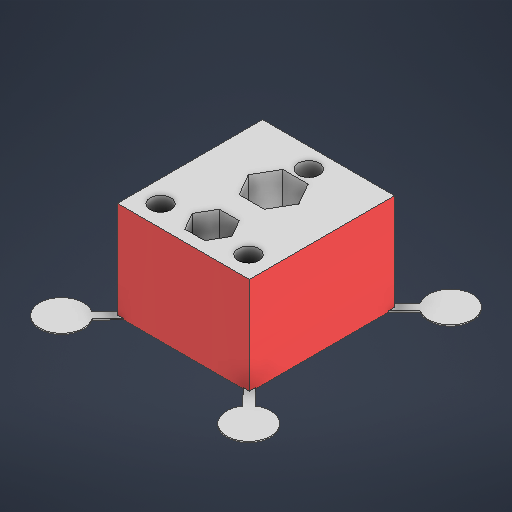
# Autodesk Inventor part: adapter-optical
Saved by Autodesk Inventor 2026.2 (Build 302298000, 298)
## iProperties
Created: 2026-05-22
Part Number: adapter-optical
Material: Generic
Document SubType Name: Modeling
Designer: mayhe
Density: 1 g/cm^3
Appearance: Default
Author: mayhe
Autodesk Inventor part; units mm, degrees
(part 1 of 2)
ref_plane "YZ Plane" through (0, 0, 0) normal (1, 0, 0) x (0, 1, 0)
ref_plane "XZ Plane" through (0, 0, 0) normal (0, 1, 0) x (-1, 0, 0)
ref_plane "XY Plane" through (0, 0, 0) normal (0, 0, 1) x (1, 0, 0)
sketch "Sketch1" plane through (0, 0, 0) normal (1, 0, 0) x (0, 1, 0)
  line L0 (11.125, 16.5) -> (-11.125, 16.5)
  line L1 (-11.125, 16.5) -> (-11.125, -16.5)
  line L2 (-11.125, -16.5) -> (11.125, -16.5)
  line L3 (11.125, -16.5) -> (11.125, 16.5)
  line L4 (11.125, 16.5) -> (-11.125, -16.5) construction
  line L5 (-11.125, 16.5) -> (11.125, -16.5) construction
  point P0 (0, 0)
  dimension "d0" = 22.25
  dimension "d1" = 33
  constraints: 12 end point, 2 midpoint, 2 parallel, 1 horizontal, 1 perpendicular
  measures "d0" distance of L2.end L1.end
  measures "d1" distance of L1.end L0.end
extrude "Extrusion1" add sketch "Sketch1" along normal mid plane 30
sketch "Sketch2" plane through (-15, -11.125, -16.5) normal (0, -1, 0) x (1, 0, 0)
  circle A0 centre (15, 4.5) radius 2.25
  line L0 (0, 0) -> (30, 0) projected
  circle A1 centre (25, 28.2) radius 2.25
  circle A2 centre (5, 28.2) radius 2.25
  point P0 (15, 16.5)
  dimension "d4" = 4.5
  dimension "d5" = 4.5
  dimension "d6" = 4.5
  dimension "d7" = 4.5
  dimension "d8" = 23.7
  dimension "d9" = 10
  dimension "d10" = 10
  constraints: 3 centre point, 1 horizontal alignment
  measures "d4" diameter of A0
  measures "d5" distance from line of L0 A0.centre
  measures "d6" diameter of A1
  measures "d7" diameter of A2
  measures "d8" vertical distance of A1.centre A0.centre
  measures "d9" horizontal distance of A0.centre A1.centre
  measures "d10" horizontal distance of A2.centre A0.centre
hole "Hole1" at (0, -11.125, -12) at (-10, -11.125, 11.7) at (10, -11.125, 11.7) direction (0, 1, 0) diameter 4.75 depth 22.25 tip angle 118 counterbore diameter 7.5 counterbore depth 3
sketch "Sketch4" plane through (-15, -11.125, -16.5) normal (0, -1, 0) x (1, 0, 0)
  circle A0 centre (15, 12.5) radius 2.0256
  circle A1 centre (15, 26.5) radius 2.1001
  line L0 (30, 33) -> (0, 33) projected
  point P0 (15, 16.5)
  point P1 (15, 33)
  dimension "d23" = 14
  dimension "d24" = 6.5
  constraints: 2 centre point, 1 midpoint
  measures "d23" distance of A1.centre A0.centre
  measures "d24" distance of point (15, 33) A1.centre
hole "Big Hole" at (0, -11.125, -4) direction (0, 1, 0) diameter 6.75 depth 22.25 tip angle 118
hole "Small Hole1" at (0, -11.125, 10) direction (0, 1, 0) diameter 5.75 depth 22.25 tip angle 118
sketch "Sketch5" plane through (-15, 11.125, 16.5) normal (0, 1, 0) x (1, 0, 0)
  circle A0 centre (15, 6.5) radius 2.875 projected
  circle A1 centre (15, 20.5) radius 3.375 projected
  circle A2 centre (15, 20.5) radius 4.975
  circle A3 centre (15, 6.5) radius 3.925
  line L0 (17.2661, 10.425) -> (19.5322, 6.5)
  line L1 (19.5322, 6.5) -> (17.2661, 2.575)
  line L2 (17.2661, 2.575) -> (12.7339, 2.575)
  line L3 (12.7339, 2.575) -> (10.4678, 6.5)
  line L4 (10.4678, 6.5) -> (12.7339, 10.425)
  line L5 (12.7339, 10.425) -> (17.2661, 10.425)
  line L6 (17.8723, 25.475) -> (20.7446, 20.5)
  line L7 (20.7446, 20.5) -> (17.8723, 15.525)
  line L8 (17.8723, 15.525) -> (12.1277, 15.525)
  line L9 (12.1277, 15.525) -> (9.2554, 20.5)
  line L10 (9.2554, 20.5) -> (12.1277, 25.475)
  line L11 (12.1277, 25.475) -> (17.8723, 25.475)
  point P0 (15, 16.5)
  point P1 (15, 10.425)
  point P2 (15, 25.475)
  dimension "d39" = 9.95
  dimension "d40" = 7.85
  constraints: 24 end point, 4 coincident, 2 midpoint, 2 vertical alignment, 30 other
extrude "Big nut seat" cut sketch "Sketch5" against normal blind 8.1168 contours A1 | A2 | A2 L6 L7 | A2 L11 L6 | L7 L8 A2 | A2 L10 L11 | L8 L9 A2 | A2 L9 L10
extrude "small nut seat" cut sketch "Sketch5" against normal blind 6.6168 contours A0 | A3 | A3 L0 L1 | A3 L5 L0 | L1 L2 A3 | A3 L4 L5 | L2 L3 A3 | A3 L3 L4
sketch "Sketch6" plane through (15, 11.125, -16.5) normal (0, 0, -1) x (-1, 0, 0)
  line L0 (2.368, -2.6371) -> (27.632, -2.6371) construction
  line L1 (27.632, -2.6371) -> (27.632, -19.6129) construction
  line L2 (27.632, -19.6129) -> (2.368, -19.6129) construction
  line L3 (2.368, -19.6129) -> (2.368, -2.6371) construction
  line L4 (12.625, 0) -> (17.375, 0) projected
  line L5 (15, 0) -> (15, -22.25)
  line L6 (17.875, -22.25) -> (12.125, -22.25) projected
  line L7 (30, 0) -> (0, 0) projected
  spline S0 degree 2 poles (11.0961, -2.1585) (11.269, -2.3611) (11.4617, -2.9539) (11.4617, -3.3343) knots 0 0 0 1 2 2 2
  spline S1 degree 2 poles (11.4617, -3.3343) (11.4617, -3.7048) (11.274, -4.305) (11.0961, -4.5075) knots 0 0 0 1 2 2 2
  spline S2 degree 2 poles (11.0961, -4.5075) (10.9084, -4.7199) (10.4119, -4.9225) (10.1131, -4.9225) knots 0 0 0 1 2 2 2
  spline S3 degree 2 poles (10.1131, -4.9225) (9.8043, -4.9225) (9.3103, -4.7125) (9.13, -4.5075) knots 0 0 0 1 2 2 2
  spline S4 degree 2 poles (9.13, -4.5075) (8.9546, -4.305) (8.7669, -3.7097) (8.7669, -3.3343) knots 0 0 0 1 2 2 2
  spline S5 degree 2 poles (8.7669, -3.3343) (8.7669, -2.9514) (8.9571, -2.3685) (9.1325, -2.1585) knots 0 0 0 1 2 2 2
  spline S6 degree 2 poles (9.1325, -2.1585) (9.3103, -1.956) (9.8068, -1.746) (10.1131, -1.746) knots 0 0 0 1 2 2 2
  spline S7 degree 2 poles (10.1131, -1.746) (10.4243, -1.746) (10.9232, -1.9634) (11.0961, -2.1585) knots 0 0 0 1 2 2 2
  spline S8 degree 2 poles (11.0393, -3.3343) (11.0393, -3.0329) (10.9084, -2.5661) (10.7899, -2.4129) knots 0 0 0 1 2 2 2
  spline S9 degree 2 poles (10.7899, -2.4129) (10.6688, -2.2549) (10.328, -2.0968) (10.1155, -2.0968) knots 0 0 0 1 2 2 2
  spline S10 degree 2 poles (10.1155, -2.0968) (9.8957, -2.0968) (9.5647, -2.2499) (9.4388, -2.4129) knots 0 0 0 1 2 2 2
  spline S11 degree 2 poles (9.4388, -2.4129) (9.3177, -2.5686) (9.1893, -3.0379) (9.1893, -3.3343) knots 0 0 0 1 2 2 2
  spline S12 degree 2 poles (9.1893, -3.3343) (9.1893, -3.9345) (9.6932, -4.5717) (10.1155, -4.5717) knots 0 0 0 1 2 2 2
  spline S13 degree 2 poles (10.1155, -4.5717) (10.5379, -4.5717) (11.0393, -3.9345) (11.0393, -3.3343) knots 0 0 0 1 2 2 2
  spline S14 degree 2 poles (13.7934, -3.6529) (13.7934, -4.2259) (13.2475, -4.9027) (12.8301, -4.9027) knots 0 0 0 1 2 2 2
  spline S15 degree 2 poles (12.8301, -4.9027) (12.6597, -4.9027) (12.3978, -4.8237) (12.262, -4.7422) knots 0 0 0 1 2 2 2
  line L8 (12.262, -4.7422) -> (12.262, -5.7005)
  line L9 (12.262, -5.7005) -> (11.8767, -5.7005)
  line L10 (11.8767, -5.7005) -> (11.8767, -2.571)
  line L11 (11.8767, -2.571) -> (12.262, -2.571)
  line L12 (12.262, -2.571) -> (12.262, -2.8106)
  spline S16 degree 2 poles (12.262, -2.8106) (12.4052, -2.6797) (12.756, -2.5068) (12.961, -2.5068) knots 0 0 0 1 2 2 2
  spline S17 degree 2 poles (12.961, -2.5068) (13.3537, -2.5068) (13.7934, -3.1293) (13.7934, -3.6529) knots 0 0 0 1 2 2 2
  spline S18 degree 2 poles (13.3957, -3.6974) (13.3957, -3.3046) (13.1463, -2.8724) (12.8671, -2.8724) knots 0 0 0 1 2 2 2
  spline S19 degree 2 poles (12.8671, -2.8724) (12.7041, -2.8724) (12.3978, -3.0181) (12.262, -3.1317) knots 0 0 0 1 2 2 2
  line L13 (12.262, -3.1317) -> (12.262, -4.431)
  spline S20 degree 2 poles (12.262, -4.431) (12.4127, -4.5026) (12.6275, -4.5569) (12.7659, -4.5569) knots 0 0 0 1 2 2 2
  spline S21 degree 2 poles (12.7659, -4.5569) (13.0647, -4.5569) (13.3957, -4.1173) (13.3957, -3.6974) knots 0 0 0 1 2 2 2
  spline S22 degree 2 poles (14.8851, -4.9027) (14.5715, -4.9027) (14.2182, -4.5446) (14.2182, -4.1568) knots 0 0 0 1 2 2 2
  line L14 (14.2182, -4.1568) -> (14.2182, -2.8897)
  line L15 (14.2182, -2.8897) -> (13.9589, -2.8897)
  line L16 (13.9589, -2.8897) -> (13.9589, -2.571)
  line L17 (13.9589, -2.571) -> (14.2182, -2.571)
  line L18 (14.2182, -2.571) -> (14.2182, -1.914)
  line L19 (14.2182, -1.914) -> (14.6036, -1.914)
  line L20 (14.6036, -1.914) -> (14.6036, -2.571)
  line L21 (14.6036, -2.571) -> (15.3125, -2.571)
  line L22 (15.3125, -2.571) -> (15.3125, -2.8897)
  line L23 (15.3125, -2.8897) -> (14.6036, -2.8897)
  line L24 (14.6036, -2.8897) -> (14.6036, -3.9789)
  spline S23 degree 2 poles (14.6036, -3.9789) (14.6036, -4.1518) (14.6159, -4.342) (14.6579, -4.4235) knots 0 0 0 1 2 2 2
  spline S24 degree 2 poles (14.6579, -4.4235) (14.6925, -4.4952) (14.8481, -4.5668) (14.9815, -4.5668) knots 0 0 0 1 2 2 2
  spline S25 degree 2 poles (14.9815, -4.5668) (15.0753, -4.5668) (15.2507, -4.51) (15.2902, -4.4927) knots 0 0 0 1 2 2 2
  line L25 (15.2902, -4.4927) -> (15.3125, -4.4927)
  line L26 (15.3125, -4.4927) -> (15.3125, -4.8385)
  spline S26 degree 2 poles (15.3125, -4.8385) (15.2038, -4.8681) (14.9815, -4.9027) (14.8851, -4.9027) knots 0 0 0 1 2 2 2
  line L27 (15.9892, -4.8583) -> (15.6039, -4.8583)
  line L28 (15.6039, -4.8583) -> (15.6039, -2.571)
  line L29 (15.6039, -2.571) -> (15.9892, -2.571)
  line L30 (15.9892, -2.571) -> (15.9892, -4.8583)
  line L31 (16.0164, -2.1906) -> (15.5792, -2.1906)
  line L32 (15.5792, -2.1906) -> (15.5792, -1.7905)
  line L33 (15.5792, -1.7905) -> (16.0164, -1.7905)
  line L34 (16.0164, -1.7905) -> (16.0164, -2.1906)
  spline S27 degree 2 poles (17.4638, -4.9101) (17.2267, -4.9101) (16.834, -4.7644) (16.6932, -4.6162) knots 0 0 0 1 2 2 2
  spline S28 degree 2 poles (16.6932, -4.6162) (16.5524, -4.4705) (16.3968, -4.0209) (16.3968, -3.7196) knots 0 0 0 1 2 2 2
  spline S29 degree 2 poles (16.3968, -3.7196) (16.3968, -3.4182) (16.5573, -2.9786) (16.6932, -2.8304) knots 0 0 0 1 2 2 2
  spline S30 degree 2 poles (16.6932, -2.8304) (16.829, -2.6797) (17.2317, -2.5192) (17.4638, -2.5192) knots 0 0 0 1 2 2 2
  spline S31 degree 2 poles (17.4638, -2.5192) (17.6516, -2.5192) (18.0023, -2.6254) (18.1382, -2.6945) knots 0 0 0 1 2 2 2
  line L35 (18.1382, -2.6945) -> (18.1382, -3.1268)
  line L36 (18.1382, -3.1268) -> (18.1159, -3.1268)
  spline S32 degree 2 poles (18.1159, -3.1268) (18.0739, -3.0922) (17.9455, -3.0033) (17.8541, -2.9564) knots 0 0 0 1 2 2 2
  spline S33 degree 2 poles (17.8541, -2.9564) (17.7726, -2.9168) (17.5552, -2.8551) (17.4564, -2.8551) knots 0 0 0 1 2 2 2
  spline S34 degree 2 poles (17.4564, -2.8551) (17.1576, -2.8551) (16.7945, -3.3071) (16.7945, -3.7196) knots 0 0 0 1 2 2 2
  spline S35 degree 2 poles (16.7945, -3.7196) (16.7945, -4.1222) (17.1452, -4.5742) (17.4564, -4.5742) knots 0 0 0 1 2 2 2
  spline S36 degree 2 poles (17.4564, -4.5742) (17.6442, -4.5742) (17.985, -4.4186) (18.1159, -4.2976) knots 0 0 0 1 2 2 2
  line L37 (18.1159, -4.2976) -> (18.1382, -4.2976)
  line L38 (18.1382, -4.2976) -> (18.1382, -4.7298)
  spline S37 degree 2 poles (18.1382, -4.7298) (18.0813, -4.757) (17.9084, -4.8336) (17.8393, -4.8509) knots 0 0 0 1 2 2 2
  spline S38 degree 2 poles (17.8393, -4.8509) (17.7405, -4.8805) (17.5849, -4.9101) (17.4638, -4.9101) knots 0 0 0 1 2 2 2
  spline S39 degree 2 poles (19.7634, -4.6162) (19.7165, -4.6508) (19.5584, -4.7743) (19.4843, -4.8113) knots 0 0 0 1 2 2 2
  spline S40 degree 2 poles (19.4843, -4.8113) (19.383, -4.8657) (19.1929, -4.9225) (19.02, -4.9225) knots 0 0 0 1 2 2 2
  spline S41 degree 2 poles (19.02, -4.9225) (18.8792, -4.9225) (18.6247, -4.8163) (18.5284, -4.7199) knots 0 0 0 1 2 2 2
  spline S42 degree 2 poles (18.5284, -4.7199) (18.437, -4.6261) (18.3259, -4.3494) (18.3259, -4.1963) knots 0 0 0 1 2 2 2
  spline S43 degree 2 poles (18.3259, -4.1963) (18.3259, -3.9592) (18.5259, -3.6233) (18.7433, -3.5269) knots 0 0 0 1 2 2 2
  spline S44 degree 2 poles (18.7433, -3.5269) (18.936, -3.438) (19.4596, -3.3713) (19.7634, -3.354) knots 0 0 0 1 2 2 2
  line L39 (19.7634, -3.354) -> (19.7634, -3.2799)
  spline S45 degree 2 poles (19.7634, -3.2799) (19.7634, -3.1465) (19.6819, -2.9811) (19.6078, -2.9341) knots 0 0 0 1 2 2 2
  spline S46 degree 2 poles (19.6078, -2.9341) (19.5337, -2.8872) (19.3213, -2.8576) (19.2077, -2.8576) knots 0 0 0 1 2 2 2
  spline S47 degree 2 poles (19.2077, -2.8576) (19.0743, -2.8576) (18.7137, -2.9366) (18.5334, -3.0132) knots 0 0 0 1 2 2 2
  line L40 (18.5334, -3.0132) -> (18.5111, -3.0132)
  line L41 (18.5111, -3.0132) -> (18.5111, -2.6204)
  spline S48 degree 2 poles (18.5111, -2.6204) (18.6173, -2.5908) (19.015, -2.5167) (19.2101, -2.5167) knots 0 0 0 1 2 2 2
  spline S49 degree 2 poles (19.2101, -2.5167) (19.4473, -2.5167) (19.7708, -2.5908) (19.8993, -2.6871) knots 0 0 0 1 2 2 2
  spline S50 degree 2 poles (19.8993, -2.6871) (20.0252, -2.781) (20.1487, -3.0799) (20.1487, -3.2947) knots 0 0 0 1 2 2 2
  line L42 (20.1487, -3.2947) -> (20.1487, -4.8583)
  line L43 (20.1487, -4.8583) -> (19.7634, -4.8583)
  line L44 (19.7634, -4.8583) -> (19.7634, -4.6162)
  line L45 (19.7634, -4.2951) -> (19.7634, -3.6603)
  spline S51 degree 2 poles (19.7634, -3.6603) (19.6251, -3.6727) (19.2077, -3.7146) (19.0768, -3.7542) knots 0 0 0 1 2 2 2
  spline S52 degree 2 poles (19.0768, -3.7542) (18.9236, -3.8011) (18.7235, -3.9962) (18.7235, -4.1691) knots 0 0 0 1 2 2 2
  spline S53 degree 2 poles (18.7235, -4.1691) (18.7235, -4.3667) (18.9459, -4.5668) (19.1583, -4.5668) knots 0 0 0 1 2 2 2
  spline S54 degree 2 poles (19.1583, -4.5668) (19.3386, -4.5668) (19.635, -4.4112) (19.7634, -4.2951) knots 0 0 0 1 2 2 2
  line L46 (21.0824, -4.8583) -> (20.6971, -4.8583)
  line L47 (20.6971, -4.8583) -> (20.6971, -1.6744)
  line L48 (20.6971, -1.6744) -> (21.0824, -1.6744)
  line L49 (21.0824, -1.6744) -> (21.0824, -4.8583)
  spline S55 degree 2 poles (9.4215, -9.9311) (9.1251, -9.9311) (8.6237, -9.731) (8.4409, -9.5309) knots 0 0 0 1 2 2 2
  spline S56 degree 2 poles (8.4409, -9.5309) (8.2581, -9.3333) (8.058, -8.7405) (8.058, -8.3552) knots 0 0 0 1 2 2 2
  spline S57 degree 2 poles (8.058, -8.3552) (8.058, -7.9723) (8.2532, -7.4042) (8.4384, -7.1943) knots 0 0 0 1 2 2 2
  spline S58 degree 2 poles (8.4384, -7.1943) (8.6212, -6.9893) (9.1201, -6.7744) (9.4289, -6.7744) knots 0 0 0 1 2 2 2
  spline S59 degree 2 poles (9.4289, -6.7744) (9.582, -6.7744) (9.8513, -6.8188) (9.9649, -6.8534) knots 0 0 0 1 2 2 2
  spline S60 degree 2 poles (9.9649, -6.8534) (10.0637, -6.8855) (10.2687, -6.9769) (10.37, -7.0313) knots 0 0 0 1 2 2 2
  line L50 (10.37, -7.0313) -> (10.37, -7.5203)
  line L51 (10.37, -7.5203) -> (10.3378, -7.5203)
  spline S61 degree 2 poles (10.3378, -7.5203) (10.2835, -7.4709) (10.1155, -7.3326) (9.9945, -7.2659) knots 0 0 0 1 2 2 2
  spline S62 degree 2 poles (9.9945, -7.2659) (9.8784, -7.2017) (9.6042, -7.1202) (9.4264, -7.1202) knots 0 0 0 1 2 2 2
  spline S63 degree 2 poles (9.4264, -7.1202) (9.2313, -7.1202) (8.883, -7.2807) (8.7521, -7.4339) knots 0 0 0 1 2 2 2
  spline S64 degree 2 poles (8.7521, -7.4339) (8.6237, -7.5895) (8.4804, -8.0613) (8.4804, -8.3552) knots 0 0 0 1 2 2 2
  spline S65 degree 2 poles (8.4804, -8.3552) (8.4804, -8.6689) (8.6311, -9.1209) (8.762, -9.2765) knots 0 0 0 1 2 2 2
  spline S66 degree 2 poles (8.762, -9.2765) (8.8904, -9.4272) (9.2337, -9.5803) (9.4264, -9.5803) knots 0 0 0 1 2 2 2
  spline S67 degree 2 poles (9.4264, -9.5803) (9.6018, -9.5803) (9.9007, -9.4939) (10.0167, -9.4296) knots 0 0 0 1 2 2 2
  spline S68 degree 2 poles (10.0167, -9.4296) (10.1279, -9.3654) (10.2934, -9.232) (10.3403, -9.1851) knots 0 0 0 1 2 2 2
  line L52 (10.3403, -9.1851) -> (10.37, -9.1851)
  line L53 (10.37, -9.1851) -> (10.37, -9.6692)
  spline S69 degree 2 poles (10.37, -9.6692) (10.2687, -9.7162) (10.0908, -9.8026) (9.9649, -9.8421) knots 0 0 0 1 2 2 2
  spline S70 degree 2 poles (9.9649, -9.8421) (9.8315, -9.8866) (9.6042, -9.9311) (9.4215, -9.9311) knots 0 0 0 1 2 2 2
  spline S71 degree 2 poles (11.9928, -9.6347) (11.9458, -9.6692) (11.7877, -9.7927) (11.7136, -9.8298) knots 0 0 0 1 2 2 2
  spline S72 degree 2 poles (11.7136, -9.8298) (11.6124, -9.8841) (11.4222, -9.9409) (11.2493, -9.9409) knots 0 0 0 1 2 2 2
  spline S73 degree 2 poles (11.2493, -9.9409) (11.1085, -9.9409) (10.8541, -9.8347) (10.7577, -9.7384) knots 0 0 0 1 2 2 2
  spline S74 degree 2 poles (10.7577, -9.7384) (10.6664, -9.6445) (10.5552, -9.3679) (10.5552, -9.2148) knots 0 0 0 1 2 2 2
  spline S75 degree 2 poles (10.5552, -9.2148) (10.5552, -8.9776) (10.7553, -8.6417) (10.9726, -8.5454) knots 0 0 0 1 2 2 2
  spline S76 degree 2 poles (10.9726, -8.5454) (11.1653, -8.4565) (11.6889, -8.3898) (11.9928, -8.3725) knots 0 0 0 1 2 2 2
  line L54 (11.9928, -8.3725) -> (11.9928, -8.2984)
  spline S77 degree 2 poles (11.9928, -8.2984) (11.9928, -8.165) (11.9112, -7.9995) (11.8371, -7.9526) knots 0 0 0 1 2 2 2
  spline S78 degree 2 poles (11.8371, -7.9526) (11.763, -7.9056) (11.5506, -7.876) (11.437, -7.876) knots 0 0 0 1 2 2 2
  spline S79 degree 2 poles (11.437, -7.876) (11.3036, -7.876) (10.943, -7.955) (10.7627, -8.0316) knots 0 0 0 1 2 2 2
  line L55 (10.7627, -8.0316) -> (10.7405, -8.0316)
  line L56 (10.7405, -8.0316) -> (10.7405, -7.6389)
  spline S80 degree 2 poles (10.7405, -7.6389) (10.8467, -7.6092) (11.2443, -7.5351) (11.4395, -7.5351) knots 0 0 0 1 2 2 2
  spline S81 degree 2 poles (11.4395, -7.5351) (11.6766, -7.5351) (12.0002, -7.6092) (12.1286, -7.7056) knots 0 0 0 1 2 2 2
  spline S82 degree 2 poles (12.1286, -7.7056) (12.2546, -7.7994) (12.3781, -8.0983) (12.3781, -8.3132) knots 0 0 0 1 2 2 2
  line L57 (12.3781, -8.3132) -> (12.3781, -9.8767)
  line L58 (12.3781, -9.8767) -> (11.9928, -9.8767)
  line L59 (11.9928, -9.8767) -> (11.9928, -9.6347)
  line L60 (11.9928, -9.3136) -> (11.9928, -8.6788)
  spline S83 degree 2 poles (11.9928, -8.6788) (11.8544, -8.6911) (11.437, -8.7331) (11.3061, -8.7726) knots 0 0 0 1 2 2 2
  spline S84 degree 2 poles (11.3061, -8.7726) (11.1529, -8.8196) (10.9529, -9.0147) (10.9529, -9.1876) knots 0 0 0 1 2 2 2
  spline S85 degree 2 poles (10.9529, -9.1876) (10.9529, -9.3852) (11.1752, -9.5853) (11.3876, -9.5853) knots 0 0 0 1 2 2 2
  spline S86 degree 2 poles (11.3876, -9.5853) (11.5679, -9.5853) (11.8643, -9.4296) (11.9928, -9.3136) knots 0 0 0 1 2 2 2
  line L61 (15.5125, -9.8767) -> (15.5125, -8.5528)
  spline S87 degree 2 poles (15.5125, -8.5528) (15.5125, -8.3947) (15.4878, -8.1255) (15.4483, -8.0514) knots 0 0 0 1 2 2 2
  spline S88 degree 2 poles (15.4483, -8.0514) (15.4088, -7.9699) (15.2581, -7.8908) (15.1272, -7.8908) knots 0 0 0 1 2 2 2
  spline S89 degree 2 poles (15.1272, -7.8908) (15.0086, -7.8908) (14.7369, -8.0366) (14.5937, -8.1749) knots 0 0 0 1 2 2 2
  spline S90 degree 2 poles (14.5937, -8.1749) (14.5962, -8.2095) (14.6011, -8.3058) (14.6011, -8.37) knots 0 0 0 1 2 2 2
  line L62 (14.6011, -8.37) -> (14.6011, -9.8767)
  line L63 (14.6011, -9.8767) -> (14.2158, -9.8767)
  line L64 (14.2158, -9.8767) -> (14.2158, -8.5528)
  spline S91 degree 2 poles (14.2158, -8.5528) (14.2158, -8.3947) (14.1911, -8.1255) (14.1515, -8.0514) knots 0 0 0 1 2 2 2
  spline S92 degree 2 poles (14.1515, -8.0514) (14.112, -7.9699) (13.9614, -7.8908) (13.8304, -7.8908) knots 0 0 0 1 2 2 2
  spline S93 degree 2 poles (13.8304, -7.8908) (13.7069, -7.8908) (13.4328, -8.0464) (13.3043, -8.1675) knots 0 0 0 1 2 2 2
  line L65 (13.3043, -8.1675) -> (13.3043, -9.8767)
  line L66 (13.3043, -9.8767) -> (12.919, -9.8767)
  line L67 (12.919, -9.8767) -> (12.919, -7.5895)
  line L68 (12.919, -7.5895) -> (13.3043, -7.5895)
  line L69 (13.3043, -7.5895) -> (13.3043, -7.8414)
  spline S94 degree 2 poles (13.3043, -7.8414) (13.455, -7.6908) (13.7514, -7.5253) (13.9292, -7.5253) knots 0 0 0 1 2 2 2
  spline S95 degree 2 poles (13.9292, -7.5253) (14.1318, -7.5253) (14.4455, -7.7105) (14.527, -7.9205) knots 0 0 0 1 2 2 2
  spline S96 degree 2 poles (14.527, -7.9205) (14.7024, -7.7253) (15.0333, -7.5253) (15.226, -7.5253) knots 0 0 0 1 2 2 2
  spline S97 degree 2 poles (15.226, -7.5253) (15.3742, -7.5253) (15.6163, -7.6167) (15.7052, -7.7204) knots 0 0 0 1 2 2 2
  spline S98 degree 2 poles (15.7052, -7.7204) (15.7966, -7.8241) (15.8979, -8.1354) (15.8979, -8.37) knots 0 0 0 1 2 2 2
  line L70 (15.8979, -8.37) -> (15.8979, -9.8767)
  line L71 (15.8979, -9.8767) -> (15.5125, -9.8767)
  spline S99 degree 2 poles (17.4317, -9.9286) (16.8834, -9.9286) (16.2807, -9.3136) (16.2807, -8.7454) knots 0 0 0 1 2 2 2
  spline S100 degree 2 poles (16.2807, -8.7454) (16.2807, -8.1872) (16.8661, -7.5253) (17.3379, -7.5253) knots 0 0 0 1 2 2 2
  spline S101 degree 2 poles (17.3379, -7.5253) (17.5503, -7.5253) (17.8788, -7.6488) (17.9998, -7.7797) knots 0 0 0 1 2 2 2
  spline S102 degree 2 poles (17.9998, -7.7797) (18.1233, -7.9106) (18.2542, -8.2885) (18.2542, -8.5627) knots 0 0 0 1 2 2 2
  line L72 (18.2542, -8.5627) -> (18.2542, -8.7726)
  line L73 (18.2542, -8.7726) -> (16.671, -8.7726)
  spline S103 degree 2 poles (16.671, -8.7726) (16.671, -9.1703) (17.0711, -9.5927) (17.4268, -9.5927) knots 0 0 0 1 2 2 2
  spline S104 degree 2 poles (17.4268, -9.5927) (17.5528, -9.5927) (17.7973, -9.5359) (17.8961, -9.4914) knots 0 0 0 1 2 2 2
  spline S105 degree 2 poles (17.8961, -9.4914) (17.9998, -9.442) (18.1431, -9.3555) (18.19, -9.316) knots 0 0 0 1 2 2 2
  line L74 (18.19, -9.316) -> (18.2123, -9.316)
  line L75 (18.2123, -9.316) -> (18.2123, -9.7359)
  spline S106 degree 2 poles (18.2123, -9.7359) (18.1456, -9.7631) (17.943, -9.8421) (17.864, -9.8644) knots 0 0 0 1 2 2 2
  spline S107 degree 2 poles (17.864, -9.8644) (17.7528, -9.8965) (17.5701, -9.9286) (17.4317, -9.9286) knots 0 0 0 1 2 2 2
  spline S108 degree 2 poles (17.8788, -8.4787) (17.8739, -8.3231) (17.8096, -8.0958) (17.7479, -8.0193) knots 0 0 0 1 2 2 2
  spline S109 degree 2 poles (17.7479, -8.0193) (17.6812, -7.9328) (17.4713, -7.8414) (17.3156, -7.8414) knots 0 0 0 1 2 2 2
  spline S110 degree 2 poles (17.3156, -7.8414) (17.1625, -7.8414) (16.9476, -7.9328) (16.8587, -8.0217) knots 0 0 0 1 2 2 2
  spline S111 degree 2 poles (16.8587, -8.0217) (16.7722, -8.1131) (16.6833, -8.333) (16.671, -8.4787) knots 0 0 0 1 2 2 2
  line L76 (16.671, -8.4787) -> (17.8788, -8.4787)
  line L77 (19.8573, -8.002) -> (19.8375, -8.002)
  spline S112 degree 2 poles (19.8375, -8.002) (19.7931, -7.9896) (19.6967, -7.9847) (19.63, -7.9847) knots 0 0 0 1 2 2 2
  spline S113 degree 2 poles (19.63, -7.9847) (19.4744, -7.9847) (19.1682, -8.1205) (19.0298, -8.2539) knots 0 0 0 1 2 2 2
  line L78 (19.0298, -8.2539) -> (19.0298, -9.8767)
  line L79 (19.0298, -9.8767) -> (18.6445, -9.8767)
  line L80 (18.6445, -9.8767) -> (18.6445, -7.5895)
  line L81 (18.6445, -7.5895) -> (19.0298, -7.5895)
  line L82 (19.0298, -7.5895) -> (19.0298, -7.9303)
  spline S114 degree 2 poles (19.0298, -7.9303) (19.2398, -7.7426) (19.5535, -7.5895) (19.7017, -7.5895) knots 0 0 0 1 2 2 2
  spline S115 degree 2 poles (19.7017, -7.5895) (19.761, -7.5895) (19.8202, -7.5944) (19.8573, -7.6018) knots 0 0 0 1 2 2 2
  line L83 (19.8573, -7.6018) -> (19.8573, -8.002)
  spline S116 degree 2 poles (21.4307, -9.6347) (21.3838, -9.6692) (21.2257, -9.7927) (21.1516, -9.8298) knots 0 0 0 1 2 2 2
  spline S117 degree 2 poles (21.1516, -9.8298) (21.0503, -9.8841) (20.8601, -9.9409) (20.6872, -9.9409) knots 0 0 0 1 2 2 2
  spline S118 degree 2 poles (20.6872, -9.9409) (20.5464, -9.9409) (20.292, -9.8347) (20.1957, -9.7384) knots 0 0 0 1 2 2 2
  spline S119 degree 2 poles (20.1957, -9.7384) (20.1043, -9.6445) (19.9931, -9.3679) (19.9931, -9.2148) knots 0 0 0 1 2 2 2
  spline S120 degree 2 poles (19.9931, -9.2148) (19.9931, -8.9776) (20.1932, -8.6417) (20.4106, -8.5454) knots 0 0 0 1 2 2 2
  spline S121 degree 2 poles (20.4106, -8.5454) (20.6032, -8.4565) (21.1269, -8.3898) (21.4307, -8.3725) knots 0 0 0 1 2 2 2
  line L84 (21.4307, -8.3725) -> (21.4307, -8.2984)
  spline S122 degree 2 poles (21.4307, -8.2984) (21.4307, -8.165) (21.3492, -7.9995) (21.2751, -7.9526) knots 0 0 0 1 2 2 2
  spline S123 degree 2 poles (21.2751, -7.9526) (21.201, -7.9056) (20.9886, -7.876) (20.8749, -7.876) knots 0 0 0 1 2 2 2
  spline S124 degree 2 poles (20.8749, -7.876) (20.7416, -7.876) (20.3809, -7.955) (20.2006, -8.0316) knots 0 0 0 1 2 2 2
  line L85 (20.2006, -8.0316) -> (20.1784, -8.0316)
  line L86 (20.1784, -8.0316) -> (20.1784, -7.6389)
  spline S125 degree 2 poles (20.1784, -7.6389) (20.2846, -7.6092) (20.6823, -7.5351) (20.8774, -7.5351) knots 0 0 0 1 2 2 2
  spline S126 degree 2 poles (20.8774, -7.5351) (21.1145, -7.5351) (21.4381, -7.6092) (21.5665, -7.7056) knots 0 0 0 1 2 2 2
  spline S127 degree 2 poles (21.5665, -7.7056) (21.6925, -7.7994) (21.816, -8.0983) (21.816, -8.3132) knots 0 0 0 1 2 2 2
  line L87 (21.816, -8.3132) -> (21.816, -9.8767)
  line L88 (21.816, -9.8767) -> (21.4307, -9.8767)
  line L89 (21.4307, -9.8767) -> (21.4307, -9.6347)
  line L90 (21.4307, -9.3136) -> (21.4307, -8.6788)
  spline S128 degree 2 poles (21.4307, -8.6788) (21.2924, -8.6911) (20.8749, -8.7331) (20.744, -8.7726) knots 0 0 0 1 2 2 2
  spline S129 degree 2 poles (20.744, -8.7726) (20.5909, -8.8196) (20.3908, -9.0147) (20.3908, -9.1876) knots 0 0 0 1 2 2 2
  spline S130 degree 2 poles (20.3908, -9.1876) (20.3908, -9.3852) (20.6131, -9.5853) (20.8255, -9.5853) knots 0 0 0 1 2 2 2
  spline S131 degree 2 poles (20.8255, -9.5853) (21.0058, -9.5853) (21.3022, -9.4296) (21.4307, -9.3136) knots 0 0 0 1 2 2 2
  line L91 (7.7456, -14.8952) -> (8.7731, -11.8472)
  line L92 (8.7731, -11.8472) -> (9.272, -11.8472)
  line L93 (9.272, -11.8472) -> (10.2996, -14.8952)
  line L94 (10.2996, -14.8952) -> (9.8722, -14.8952)
  line L95 (9.8722, -14.8952) -> (9.5956, -14.043)
  line L96 (9.5956, -14.043) -> (8.4322, -14.043)
  line L97 (8.4322, -14.043) -> (8.1556, -14.8952)
  line L98 (8.1556, -14.8952) -> (7.7456, -14.8952)
  line L99 (9.4845, -13.6972) -> (9.0127, -12.2621)
  line L100 (9.0127, -12.2621) -> (8.5434, -13.6972)
  line L101 (8.5434, -13.6972) -> (9.4845, -13.6972)
  line L102 (12.3176, -14.8952) -> (11.9322, -14.8952)
  line L103 (11.9322, -14.8952) -> (11.9322, -14.663)
  spline S132 degree 2 poles (11.9322, -14.663) (11.8433, -14.7371) (11.7124, -14.8359) (11.6235, -14.8779) knots 0 0 0 1 2 2 2
  spline S133 degree 2 poles (11.6235, -14.8779) (11.542, -14.9174) (11.3666, -14.9594) (11.2505, -14.9594) knots 0 0 0 1 2 2 2
  spline S134 degree 2 poles (11.2505, -14.9594) (11.0628, -14.9594) (10.7466, -14.8038) (10.6355, -14.6531) knots 0 0 0 1 2 2 2
  spline S135 degree 2 poles (10.6355, -14.6531) (10.5243, -14.5024) (10.4008, -14.0578) (10.4008, -13.7688) knots 0 0 0 1 2 2 2
  spline S136 degree 2 poles (10.4008, -13.7688) (10.4008, -13.4675) (10.5564, -13.0278) (10.6923, -12.8623) knots 0 0 0 1 2 2 2
  spline S137 degree 2 poles (10.6923, -12.8623) (10.8183, -12.7141) (11.1715, -12.5437) (11.3666, -12.5437) knots 0 0 0 1 2 2 2
  spline S138 degree 2 poles (11.3666, -12.5437) (11.537, -12.5437) (11.7914, -12.6203) (11.9322, -12.6993) knots 0 0 0 1 2 2 2
  line L104 (11.9322, -12.6993) -> (11.9322, -11.7113)
  line L105 (11.9322, -11.7113) -> (12.3176, -11.7113)
  line L106 (12.3176, -11.7113) -> (12.3176, -14.8952)
  line L107 (11.9322, -14.3394) -> (11.9322, -13.018)
  spline S139 degree 2 poles (11.9322, -13.018) (11.789, -12.9488) (11.5617, -12.8969) (11.4308, -12.8969) knots 0 0 0 1 2 2 2
  spline S140 degree 2 poles (11.4308, -12.8969) (11.1344, -12.8969) (10.7985, -13.3415) (10.7985, -13.7614) knots 0 0 0 1 2 2 2
  spline S141 degree 2 poles (10.7985, -13.7614) (10.7985, -14.1665) (11.0554, -14.5938) (11.3394, -14.5938) knots 0 0 0 1 2 2 2
  spline S142 degree 2 poles (11.3394, -14.5938) (11.4901, -14.5938) (11.7964, -14.4555) (11.9322, -14.3394) knots 0 0 0 1 2 2 2
  spline S143 degree 2 poles (14.1503, -14.6531) (14.1034, -14.6877) (13.9453, -14.8112) (13.8712, -14.8482) knots 0 0 0 1 2 2 2
  spline S144 degree 2 poles (13.8712, -14.8482) (13.7699, -14.9026) (13.5797, -14.9594) (13.4068, -14.9594) knots 0 0 0 1 2 2 2
  spline S145 degree 2 poles (13.4068, -14.9594) (13.266, -14.9594) (13.0116, -14.8532) (12.9153, -14.7568) knots 0 0 0 1 2 2 2
  spline S146 degree 2 poles (12.9153, -14.7568) (12.8239, -14.663) (12.7128, -14.3863) (12.7128, -14.2332) knots 0 0 0 1 2 2 2
  spline S147 degree 2 poles (12.7128, -14.2332) (12.7128, -13.9961) (12.9128, -13.6602) (13.1302, -13.5638) knots 0 0 0 1 2 2 2
  spline S148 degree 2 poles (13.1302, -13.5638) (13.3229, -13.4749) (13.8465, -13.4082) (14.1503, -13.3909) knots 0 0 0 1 2 2 2
  line L108 (14.1503, -13.3909) -> (14.1503, -13.3168)
  spline S149 degree 2 poles (14.1503, -13.3168) (14.1503, -13.1834) (14.0688, -13.018) (13.9947, -12.971) knots 0 0 0 1 2 2 2
  spline S150 degree 2 poles (13.9947, -12.971) (13.9206, -12.9241) (13.7082, -12.8945) (13.5946, -12.8945) knots 0 0 0 1 2 2 2
  spline S151 degree 2 poles (13.5946, -12.8945) (13.4612, -12.8945) (13.1006, -12.9735) (12.9202, -13.0501) knots 0 0 0 1 2 2 2
  line L109 (12.9202, -13.0501) -> (12.898, -13.0501)
  line L110 (12.898, -13.0501) -> (12.898, -12.6573)
  spline S152 degree 2 poles (12.898, -12.6573) (13.0042, -12.6277) (13.4019, -12.5536) (13.597, -12.5536) knots 0 0 0 1 2 2 2
  spline S153 degree 2 poles (13.597, -12.5536) (13.8342, -12.5536) (14.1577, -12.6277) (14.2862, -12.724) knots 0 0 0 1 2 2 2
  spline S154 degree 2 poles (14.2862, -12.724) (14.4121, -12.8179) (14.5356, -13.1168) (14.5356, -13.3316) knots 0 0 0 1 2 2 2
  line L111 (14.5356, -13.3316) -> (14.5356, -14.8952)
  line L112 (14.5356, -14.8952) -> (14.1503, -14.8952)
  line L113 (14.1503, -14.8952) -> (14.1503, -14.6531)
  line L114 (14.1503, -14.332) -> (14.1503, -13.6972)
  spline S155 degree 2 poles (14.1503, -13.6972) (14.012, -13.7096) (13.5946, -13.7516) (13.4636, -13.7911) knots 0 0 0 1 2 2 2
  spline S156 degree 2 poles (13.4636, -13.7911) (13.3105, -13.838) (13.1104, -14.0331) (13.1104, -14.206) knots 0 0 0 1 2 2 2
  spline S157 degree 2 poles (13.1104, -14.206) (13.1104, -14.4036) (13.3327, -14.6037) (13.5452, -14.6037) knots 0 0 0 1 2 2 2
  spline S158 degree 2 poles (13.5452, -14.6037) (13.7255, -14.6037) (14.0219, -14.4481) (14.1503, -14.332) knots 0 0 0 1 2 2 2
  spline S159 degree 2 poles (16.9933, -13.6898) (16.9933, -14.2628) (16.4474, -14.9396) (16.03, -14.9396) knots 0 0 0 1 2 2 2
  spline S160 degree 2 poles (16.03, -14.9396) (15.8596, -14.9396) (15.5977, -14.8606) (15.4619, -14.7791) knots 0 0 0 1 2 2 2
  line L115 (15.4619, -14.7791) -> (15.4619, -15.7374)
  line L116 (15.4619, -15.7374) -> (15.0766, -15.7374)
  line L117 (15.0766, -15.7374) -> (15.0766, -12.6079)
  line L118 (15.0766, -12.6079) -> (15.4619, -12.6079)
  line L119 (15.4619, -12.6079) -> (15.4619, -12.8475)
  spline S161 degree 2 poles (15.4619, -12.8475) (15.6052, -12.7166) (15.9559, -12.5437) (16.1609, -12.5437) knots 0 0 0 1 2 2 2
  spline S162 degree 2 poles (16.1609, -12.5437) (16.5536, -12.5437) (16.9933, -13.1662) (16.9933, -13.6898) knots 0 0 0 1 2 2 2
  spline S163 degree 2 poles (16.5956, -13.7343) (16.5956, -13.3415) (16.3462, -12.9093) (16.067, -12.9093) knots 0 0 0 1 2 2 2
  spline S164 degree 2 poles (16.067, -12.9093) (15.904, -12.9093) (15.5977, -13.055) (15.4619, -13.1686) knots 0 0 0 1 2 2 2
  line L120 (15.4619, -13.1686) -> (15.4619, -14.4679)
  spline S165 degree 2 poles (15.4619, -14.4679) (15.6126, -14.5395) (15.8275, -14.5938) (15.9658, -14.5938) knots 0 0 0 1 2 2 2
  spline S166 degree 2 poles (15.9658, -14.5938) (16.2646, -14.5938) (16.5956, -14.1542) (16.5956, -13.7343) knots 0 0 0 1 2 2 2
  spline S167 degree 2 poles (18.0851, -14.9396) (17.7714, -14.9396) (17.4181, -14.5815) (17.4181, -14.1937) knots 0 0 0 1 2 2 2
  line L121 (17.4181, -14.1937) -> (17.4181, -12.9266)
  line L122 (17.4181, -12.9266) -> (17.1588, -12.9266)
  line L123 (17.1588, -12.9266) -> (17.1588, -12.6079)
  line L124 (17.1588, -12.6079) -> (17.4181, -12.6079)
  line L125 (17.4181, -12.6079) -> (17.4181, -11.9509)
  line L126 (17.4181, -11.9509) -> (17.8035, -11.9509)
  line L127 (17.8035, -11.9509) -> (17.8035, -12.6079)
  line L128 (17.8035, -12.6079) -> (18.5124, -12.6079)
  line L129 (18.5124, -12.6079) -> (18.5124, -12.9266)
  line L130 (18.5124, -12.9266) -> (17.8035, -12.9266)
  line L131 (17.8035, -12.9266) -> (17.8035, -14.0158)
  spline S168 degree 2 poles (17.8035, -14.0158) (17.8035, -14.1887) (17.8158, -14.3789) (17.8578, -14.4604) knots 0 0 0 1 2 2 2
  spline S169 degree 2 poles (17.8578, -14.4604) (17.8924, -14.5321) (18.048, -14.6037) (18.1814, -14.6037) knots 0 0 0 1 2 2 2
  spline S170 degree 2 poles (18.1814, -14.6037) (18.2752, -14.6037) (18.4506, -14.5469) (18.4901, -14.5296) knots 0 0 0 1 2 2 2
  line L132 (18.4901, -14.5296) -> (18.5124, -14.5296)
  line L133 (18.5124, -14.5296) -> (18.5124, -14.8754)
  spline S171 degree 2 poles (18.5124, -14.8754) (18.4037, -14.905) (18.1814, -14.9396) (18.0851, -14.9396) knots 0 0 0 1 2 2 2
  spline S172 degree 2 poles (19.7894, -14.947) (19.241, -14.947) (18.6383, -14.332) (18.6383, -13.7639) knots 0 0 0 1 2 2 2
  spline S173 degree 2 poles (18.6383, -13.7639) (18.6383, -13.2057) (19.2237, -12.5437) (19.6955, -12.5437) knots 0 0 0 1 2 2 2
  spline S174 degree 2 poles (19.6955, -12.5437) (19.9079, -12.5437) (20.2364, -12.6672) (20.3575, -12.7981) knots 0 0 0 1 2 2 2
  spline S175 degree 2 poles (20.3575, -12.7981) (20.481, -12.929) (20.6119, -13.3069) (20.6119, -13.5811) knots 0 0 0 1 2 2 2
  line L134 (20.6119, -13.5811) -> (20.6119, -13.7911)
  line L135 (20.6119, -13.7911) -> (19.0286, -13.7911)
  spline S176 degree 2 poles (19.0286, -13.7911) (19.0286, -14.1887) (19.4287, -14.6111) (19.7844, -14.6111) knots 0 0 0 1 2 2 2
  spline S177 degree 2 poles (19.7844, -14.6111) (19.9104, -14.6111) (20.1549, -14.5543) (20.2537, -14.5098) knots 0 0 0 1 2 2 2
  spline S178 degree 2 poles (20.2537, -14.5098) (20.3575, -14.4604) (20.5007, -14.374) (20.5477, -14.3345) knots 0 0 0 1 2 2 2
  line L136 (20.5477, -14.3345) -> (20.5699, -14.3345)
  line L137 (20.5699, -14.3345) -> (20.5699, -14.7544)
  spline S179 degree 2 poles (20.5699, -14.7544) (20.5032, -14.7815) (20.3007, -14.8606) (20.2216, -14.8828) knots 0 0 0 1 2 2 2
  spline S180 degree 2 poles (20.2216, -14.8828) (20.1105, -14.9149) (19.9277, -14.947) (19.7894, -14.947) knots 0 0 0 1 2 2 2
  spline S181 degree 2 poles (20.2364, -13.4971) (20.2315, -13.3415) (20.1673, -13.1143) (20.1055, -13.0377) knots 0 0 0 1 2 2 2
  spline S182 degree 2 poles (20.1055, -13.0377) (20.0388, -12.9513) (19.8289, -12.8599) (19.6733, -12.8599) knots 0 0 0 1 2 2 2
  spline S183 degree 2 poles (19.6733, -12.8599) (19.5201, -12.8599) (19.3052, -12.9513) (19.2163, -13.0402) knots 0 0 0 1 2 2 2
  spline S184 degree 2 poles (19.2163, -13.0402) (19.1299, -13.1316) (19.0409, -13.3514) (19.0286, -13.4971) knots 0 0 0 1 2 2 2
  line L138 (19.0286, -13.4971) -> (20.2364, -13.4971)
  line L139 (22.2149, -13.0204) -> (22.1952, -13.0204)
  spline S185 degree 2 poles (22.1952, -13.0204) (22.1507, -13.0081) (22.0544, -13.0031) (21.9877, -13.0031) knots 0 0 0 1 2 2 2
  spline S186 degree 2 poles (21.9877, -13.0031) (21.8321, -13.0031) (21.5258, -13.139) (21.3875, -13.2724) knots 0 0 0 1 2 2 2
  line L140 (21.3875, -13.2724) -> (21.3875, -14.8952)
  line L141 (21.3875, -14.8952) -> (21.0021, -14.8952)
  line L142 (21.0021, -14.8952) -> (21.0021, -12.6079)
  line L143 (21.0021, -12.6079) -> (21.3875, -12.6079)
  line L144 (21.3875, -12.6079) -> (21.3875, -12.9488)
  spline S187 degree 2 poles (21.3875, -12.9488) (21.5974, -12.7611) (21.9111, -12.6079) (22.0593, -12.6079) knots 0 0 0 1 2 2 2
  spline S188 degree 2 poles (22.0593, -12.6079) (22.1186, -12.6079) (22.1779, -12.6129) (22.2149, -12.6203) knots 0 0 0 1 2 2 2
  line L145 (22.2149, -12.6203) -> (22.2149, -13.0204)
  spline S189 degree 2 poles (7.4615, -18.9454) (7.4615, -19.1652) (7.3207, -19.5406) (7.1923, -19.679) knots 0 0 0 1 2 2 2
  spline S190 degree 2 poles (7.1923, -19.679) (7.0638, -19.8173) (6.681, -19.9778) (6.4439, -19.9778) knots 0 0 0 1 2 2 2
  spline S191 degree 2 poles (6.4439, -19.9778) (6.2265, -19.9778) (5.8017, -19.8815) (5.646, -19.8049) knots 0 0 0 1 2 2 2
  line L146 (5.646, -19.8049) -> (5.646, -19.3727)
  line L147 (5.646, -19.3727) -> (5.6757, -19.3727)
  spline S192 degree 2 poles (5.6757, -19.3727) (5.7226, -19.4073) (5.898, -19.4962) (6.0042, -19.5357) knots 0 0 0 1 2 2 2
  spline S193 degree 2 poles (6.0042, -19.5357) (6.1252, -19.5777) (6.3253, -19.6246) (6.4513, -19.6246) knots 0 0 0 1 2 2 2
  spline S194 degree 2 poles (6.4513, -19.6246) (6.5748, -19.6246) (6.807, -19.5357) (6.8909, -19.4394) knots 0 0 0 1 2 2 2
  spline S195 degree 2 poles (6.8909, -19.4394) (6.9675, -19.348) (7.0465, -19.1059) (7.0465, -18.9429) knots 0 0 0 1 2 2 2
  spline S196 degree 2 poles (7.0465, -18.9429) (7.0465, -18.7799) (6.9576, -18.5724) (6.8736, -18.5032) knots 0 0 0 1 2 2 2
  spline S197 degree 2 poles (6.8736, -18.5032) (6.7872, -18.4267) (6.5303, -18.3625) (6.3747, -18.3625) knots 0 0 0 1 2 2 2
  spline S198 degree 2 poles (6.3747, -18.3625) (6.2067, -18.3625) (5.8733, -18.4143) (5.772, -18.4366) knots 0 0 0 1 2 2 2
  line L148 (5.772, -18.4366) -> (5.772, -16.8656)
  line L149 (5.772, -16.8656) -> (7.4442, -16.8656)
  line L150 (7.4442, -16.8656) -> (7.4442, -17.2238)
  line L151 (7.4442, -17.2238) -> (6.1648, -17.2238)
  line L152 (6.1648, -17.2238) -> (6.1648, -18.0364)
  spline S199 degree 2 poles (6.1648, -18.0364) (6.2389, -18.0265) (6.3821, -18.0191) (6.4414, -18.0191) knots 0 0 0 1 2 2 2
  spline S200 degree 2 poles (6.4414, -18.0191) (6.676, -18.0191) (6.9996, -18.0957) (7.1478, -18.2093) knots 0 0 0 1 2 2 2
  spline S201 degree 2 poles (7.1478, -18.2093) (7.2985, -18.3229) (7.4615, -18.6687) (7.4615, -18.9454) knots 0 0 0 1 2 2 2
  line L153 (9.1683, -16.7298) -> (7.9753, -20.5756)
  line L154 (7.9753, -20.5756) -> (7.6295, -20.5756)
  line L155 (7.6295, -20.5756) -> (8.8175, -16.7298)
  line L156 (8.8175, -16.7298) -> (9.1683, -16.7298)
  line L157 (11.3839, -19.9136) -> (9.5042, -19.9136)
  line L158 (9.5042, -19.9136) -> (9.5042, -19.4814)
  spline S202 degree 2 poles (9.5042, -19.4814) (9.7068, -19.2912) (10.0674, -18.938) (10.2403, -18.7478) knots 0 0 0 1 2 2 2
  spline S203 degree 2 poles (10.2403, -18.7478) (10.5886, -18.3649) (10.843, -17.9055) (10.843, -17.661) knots 0 0 0 1 2 2 2
  spline S204 degree 2 poles (10.843, -17.661) (10.843, -17.5325) (10.7639, -17.3399) (10.6923, -17.2781) knots 0 0 0 1 2 2 2
  spline S205 degree 2 poles (10.6923, -17.2781) (10.6207, -17.2164) (10.4329, -17.1546) (10.3193, -17.1546) knots 0 0 0 1 2 2 2
  spline S206 degree 2 poles (10.3193, -17.1546) (10.2106, -17.1546) (9.9883, -17.209) (9.8871, -17.2509) knots 0 0 0 1 2 2 2
  spline S207 degree 2 poles (9.8871, -17.2509) (9.8006, -17.2855) (9.6401, -17.3843) (9.5907, -17.4189) knots 0 0 0 1 2 2 2
  line L159 (9.5907, -17.4189) -> (9.5684, -17.4189)
  line L160 (9.5684, -17.4189) -> (9.5684, -16.9842)
  spline S208 degree 2 poles (9.5684, -16.9842) (9.6944, -16.9224) (10.1464, -16.8014) (10.349, -16.8014) knots 0 0 0 1 2 2 2
  spline S209 degree 2 poles (10.349, -16.8014) (10.7763, -16.8014) (11.2579, -17.2534) (11.2579, -17.6387) knots 0 0 0 1 2 2 2
  spline S210 degree 2 poles (11.2579, -17.6387) (11.2579, -17.819) (11.1739, -18.1204) (11.0998, -18.2488) knots 0 0 0 1 2 2 2
  spline S211 degree 2 poles (11.0998, -18.2488) (11.0257, -18.3822) (10.8109, -18.644) (10.6923, -18.77) knots 0 0 0 1 2 2 2
  spline S212 degree 2 poles (10.6923, -18.77) (10.4996, -18.98) (10.0279, -19.4295) (9.8871, -19.5604) knots 0 0 0 1 2 2 2
  line L161 (9.8871, -19.5604) -> (11.3839, -19.5604)
  line L162 (11.3839, -19.5604) -> (11.3839, -19.9136)
  line L163 (13.7057, -17.3226) -> (12.3867, -19.9136)
  line L164 (12.3867, -19.9136) -> (11.952, -19.9136)
  line L165 (11.952, -19.9136) -> (13.3451, -17.2238)
  line L166 (13.3451, -17.2238) -> (11.7717, -17.2238)
  line L167 (11.7717, -17.2238) -> (11.7717, -16.8656)
  line L168 (11.7717, -16.8656) -> (13.7057, -16.8656)
  line L169 (13.7057, -16.8656) -> (13.7057, -17.3226)
  line L170 (15.3458, -16.7298) -> (14.1528, -20.5756)
  line L171 (14.1528, -20.5756) -> (13.807, -20.5756)
  line L172 (13.807, -20.5756) -> (14.9951, -16.7298)
  line L173 (14.9951, -16.7298) -> (15.3458, -16.7298)
  line L174 (17.5614, -19.9136) -> (15.6817, -19.9136)
  line L175 (15.6817, -19.9136) -> (15.6817, -19.4814)
  spline S213 degree 2 poles (15.6817, -19.4814) (15.8843, -19.2912) (16.2449, -18.938) (16.4178, -18.7478) knots 0 0 0 1 2 2 2
  spline S214 degree 2 poles (16.4178, -18.7478) (16.7661, -18.3649) (17.0205, -17.9055) (17.0205, -17.661) knots 0 0 0 1 2 2 2
  spline S215 degree 2 poles (17.0205, -17.661) (17.0205, -17.5325) (16.9414, -17.3399) (16.8698, -17.2781) knots 0 0 0 1 2 2 2
  spline S216 degree 2 poles (16.8698, -17.2781) (16.7982, -17.2164) (16.6105, -17.1546) (16.4968, -17.1546) knots 0 0 0 1 2 2 2
  spline S217 degree 2 poles (16.4968, -17.1546) (16.3881, -17.1546) (16.1658, -17.209) (16.0646, -17.2509) knots 0 0 0 1 2 2 2
  spline S218 degree 2 poles (16.0646, -17.2509) (15.9781, -17.2855) (15.8176, -17.3843) (15.7682, -17.4189) knots 0 0 0 1 2 2 2
  line L176 (15.7682, -17.4189) -> (15.7459, -17.4189)
  line L177 (15.7459, -17.4189) -> (15.7459, -16.9842)
  spline S219 degree 2 poles (15.7459, -16.9842) (15.8719, -16.9224) (16.3239, -16.8014) (16.5265, -16.8014) knots 0 0 0 1 2 2 2
  spline S220 degree 2 poles (16.5265, -16.8014) (16.9538, -16.8014) (17.4354, -17.2534) (17.4354, -17.6387) knots 0 0 0 1 2 2 2
  spline S221 degree 2 poles (17.4354, -17.6387) (17.4354, -17.819) (17.3515, -18.1204) (17.2774, -18.2488) knots 0 0 0 1 2 2 2
  spline S222 degree 2 poles (17.2774, -18.2488) (17.2033, -18.3822) (16.9884, -18.644) (16.8698, -18.77) knots 0 0 0 1 2 2 2
  spline S223 degree 2 poles (16.8698, -18.77) (16.6771, -18.98) (16.2054, -19.4295) (16.0646, -19.5604) knots 0 0 0 1 2 2 2
  line L178 (16.0646, -19.5604) -> (17.5614, -19.5604)
  line L179 (17.5614, -19.5604) -> (17.5614, -19.9136)
  spline S224 degree 2 poles (19.8659, -18.3896) (19.8659, -19.2097) (19.3892, -19.9778) (18.8927, -19.9778) knots 0 0 0 1 2 2 2
  spline S225 degree 2 poles (18.8927, -19.9778) (18.3889, -19.9778) (17.9171, -19.1948) (17.9171, -18.3921) knots 0 0 0 1 2 2 2
  spline S226 degree 2 poles (17.9171, -18.3921) (17.9171, -17.5671) (18.3938, -16.8039) (18.8927, -16.8039) knots 0 0 0 1 2 2 2
  spline S227 degree 2 poles (18.8927, -16.8039) (19.3942, -16.8039) (19.8659, -17.5943) (19.8659, -18.3896) knots 0 0 0 1 2 2 2
  spline S228 degree 2 poles (19.3423, -19.3183) (19.4016, -19.1677) (19.451, -18.7033) (19.451, -18.3896) knots 0 0 0 1 2 2 2
  spline S229 degree 2 poles (19.451, -18.3896) (19.451, -18.0759) (19.4016, -17.614) (19.3398, -17.4584) knots 0 0 0 1 2 2 2
  spline S230 degree 2 poles (19.3398, -17.4584) (19.2781, -17.3028) (19.0632, -17.1423) (18.8927, -17.1423) knots 0 0 0 1 2 2 2
  spline S231 degree 2 poles (18.8927, -17.1423) (18.7223, -17.1423) (18.5025, -17.3028) (18.4383, -17.4634) knots 0 0 0 1 2 2 2
  spline S232 degree 2 poles (18.4383, -17.4634) (18.3765, -17.619) (18.3321, -18.0932) (18.3321, -18.3921) knots 0 0 0 1 2 2 2
  spline S233 degree 2 poles (18.3321, -18.3921) (18.3321, -18.7132) (18.3716, -19.143) (18.4358, -19.3109) knots 0 0 0 1 2 2 2
  spline S234 degree 2 poles (18.4358, -19.3109) (18.4951, -19.469) (18.7149, -19.6394) (18.8927, -19.6394) knots 0 0 0 1 2 2 2
  spline S235 degree 2 poles (18.8927, -19.6394) (19.0607, -19.6394) (19.2805, -19.4789) (19.3423, -19.3183) knots 0 0 0 1 2 2 2
  line L180 (22.1359, -19.9136) -> (20.2562, -19.9136)
  line L181 (20.2562, -19.9136) -> (20.2562, -19.4814)
  spline S236 degree 2 poles (20.2562, -19.4814) (20.4587, -19.2912) (20.8194, -18.938) (20.9923, -18.7478) knots 0 0 0 1 2 2 2
  spline S237 degree 2 poles (20.9923, -18.7478) (21.3405, -18.3649) (21.5949, -17.9055) (21.5949, -17.661) knots 0 0 0 1 2 2 2
  spline S238 degree 2 poles (21.5949, -17.661) (21.5949, -17.5325) (21.5159, -17.3399) (21.4443, -17.2781) knots 0 0 0 1 2 2 2
  spline S239 degree 2 poles (21.4443, -17.2781) (21.3726, -17.2164) (21.1849, -17.1546) (21.0713, -17.1546) knots 0 0 0 1 2 2 2
  spline S240 degree 2 poles (21.0713, -17.1546) (20.9626, -17.1546) (20.7403, -17.209) (20.639, -17.2509) knots 0 0 0 1 2 2 2
  spline S241 degree 2 poles (20.639, -17.2509) (20.5526, -17.2855) (20.392, -17.3843) (20.3426, -17.4189) knots 0 0 0 1 2 2 2
  line L182 (20.3426, -17.4189) -> (20.3204, -17.4189)
  line L183 (20.3204, -17.4189) -> (20.3204, -16.9842)
  spline S242 degree 2 poles (20.3204, -16.9842) (20.4464, -16.9224) (20.8984, -16.8014) (21.1009, -16.8014) knots 0 0 0 1 2 2 2
  spline S243 degree 2 poles (21.1009, -16.8014) (21.5283, -16.8014) (22.0099, -17.2534) (22.0099, -17.6387) knots 0 0 0 1 2 2 2
  spline S244 degree 2 poles (22.0099, -17.6387) (22.0099, -17.819) (21.9259, -18.1204) (21.8518, -18.2488) knots 0 0 0 1 2 2 2
  spline S245 degree 2 poles (21.8518, -18.2488) (21.7777, -18.3822) (21.5628, -18.644) (21.4443, -18.77) knots 0 0 0 1 2 2 2
  spline S246 degree 2 poles (21.4443, -18.77) (21.2516, -18.98) (20.7798, -19.4295) (20.639, -19.5604) knots 0 0 0 1 2 2 2
  line L184 (20.639, -19.5604) -> (22.1359, -19.5604)
  line L185 (22.1359, -19.5604) -> (22.1359, -19.9136)
  spline S247 degree 2 poles (24.47, -18.9256) (24.47, -19.1603) (24.3144, -19.5579) (24.1835, -19.6913) knots 0 0 0 1 2 2 2
  spline S248 degree 2 poles (24.1835, -19.6913) (24.0477, -19.8321) (23.7068, -19.9778) (23.5018, -19.9778) knots 0 0 0 1 2 2 2
  spline S249 degree 2 poles (23.5018, -19.9778) (23.2968, -19.9778) (22.9584, -19.8395) (22.83, -19.7012) knots 0 0 0 1 2 2 2
  spline S250 degree 2 poles (22.83, -19.7012) (22.6719, -19.5357) (22.494, -18.98) (22.494, -18.5749) knots 0 0 0 1 2 2 2
  spline S251 degree 2 poles (22.494, -18.5749) (22.494, -18.1772) (22.6571, -17.5375) (22.8275, -17.3003) knots 0 0 0 1 2 2 2
  spline S252 degree 2 poles (22.8275, -17.3003) (22.993, -17.0682) (23.5166, -16.8088) (23.8599, -16.8088) knots 0 0 0 1 2 2 2
  spline S253 degree 2 poles (23.8599, -16.8088) (23.9612, -16.8088) (24.1391, -16.8286) (24.2058, -16.8508) knots 0 0 0 1 2 2 2
  line L186 (24.2058, -16.8508) -> (24.2058, -17.2435)
  line L187 (24.2058, -17.2435) -> (24.1885, -17.2435)
  spline S254 degree 2 poles (24.1885, -17.2435) (24.1317, -17.2139) (23.9242, -17.162) (23.8056, -17.162) knots 0 0 0 1 2 2 2
  spline S255 degree 2 poles (23.8056, -17.162) (23.4252, -17.162) (22.9584, -17.6758) (22.9139, -18.1797) knots 0 0 0 1 2 2 2
  spline S256 degree 2 poles (22.9139, -18.1797) (23.0597, -18.0784) (23.3659, -17.9672) (23.5487, -17.9672) knots 0 0 0 1 2 2 2
  spline S257 degree 2 poles (23.5487, -17.9672) (23.7266, -17.9672) (23.9933, -18.0389) (24.1391, -18.1476) knots 0 0 0 1 2 2 2
  spline S258 degree 2 poles (24.1391, -18.1476) (24.307, -18.2735) (24.47, -18.6638) (24.47, -18.9256) knots 0 0 0 1 2 2 2
  spline S259 degree 2 poles (24.0551, -18.9429) (24.0551, -18.7552) (23.9563, -18.5008) (23.8476, -18.4119) knots 0 0 0 1 2 2 2
  spline S260 degree 2 poles (23.8476, -18.4119) (23.7661, -18.3476) (23.5635, -18.3056) (23.4573, -18.3056) knots 0 0 0 1 2 2 2
  spline S261 degree 2 poles (23.4573, -18.3056) (23.3141, -18.3056) (23.0448, -18.3921) (22.9139, -18.4736) knots 0 0 0 1 2 2 2
  spline S262 degree 2 poles (22.9139, -18.4736) (22.9115, -18.5181) (22.9065, -18.602) (22.9065, -18.6663) knots 0 0 0 1 2 2 2
  spline S263 degree 2 poles (22.9065, -18.6663) (22.9065, -18.9824) (23.03, -19.3702) (23.1239, -19.4715) knots 0 0 0 1 2 2 2
  spline S264 degree 2 poles (23.1239, -19.4715) (23.2103, -19.5678) (23.3981, -19.6444) (23.5043, -19.6444) knots 0 0 0 1 2 2 2
  spline S265 degree 2 poles (23.5043, -19.6444) (23.7513, -19.6444) (24.0551, -19.2936) (24.0551, -18.9429) knots 0 0 0 1 2 2 2
  point P0 (15, -11.125)
  point P1 (27.632, -11.125)
  point P2 (15, -11.125)
  point P3 (15, -2.6371)
  point P4 (15, 0)
  dimension "d0" = 22.25
  dimension "d1" = 33
  constraints: 6 midpoint, 2 end point, 1 horizontal alignment, 1 vertical alignment, 2 other
extrude "Text" cut sketch "Sketch6" along normal mid plane 1 contours L21 L22 L23 L5 | L5 L23 L24 S23 S24 S25 S26 S22 L14 L15 L16 L17 L18 L19 L20 L21 | S25 L25 L26 S26 L5 | S96 S97 S98 L70 L71 L61 S87 S88 S89 L5 | L5 S89 S90 L62 L63 L64 S91 S92 S93 L65 L66 L67 L68 L69 S94 S95 S96 | L173 L170 L5 | L5 L170 L171 L172 L173 | S0 S1 S2 S3 S4 S5 S6 S7 | S14 S15 L8 L9 L10 L11 L12 S16 S17 | L27 L28 L29 L30 | L31 L32 L33 L34 | S27 S28 S29 S30 S31 L35 L36 S32 S33 S34 S35 S36 L37 L38 S37 S38 | S39 S40 S41 S42 S43 S44 L39 S45 S46 S47 L40 L41 S48 S49 S50 L42 L43 L44 | L46 L47 L48 L49 | S55 S56 S57 S58 S59 S60 L50 L51 S61 S62 S63 S64 S65 S66 S67 S68 L52 L53 S69 S70 | S71 S72 S73 S74 S75 S76 L54 S77 S78 S79 L55 L56 S80 S81 S82 L57 L58 L59 | S99 S100 S101 S102 L72 L73 S103 S104 S105 L74 L75 S106 S107 | L77 S112 S113 L78 L79 L80 L81 L82 S114 S115 L83 | S116 S117 S118 S119 S120 S121 L84 S122 S123 S124 L85 L86 S125 S126 S127 L87 L88 L89 | L91 L92 L93 L94 L95 L96 L97 L98 | L102 L103 S132 S133 S134 S135 S136 S137 S138 L104 L105 L106 | S143 S144 S145 S146 S147 S148 L108 S149 S150 S151 L109 L110 S152 S153 S154 L111 L112 L113 | S159 S160 L115 L116 L117 L118 L119 S161 S162 | S167 L121 L122 L123 L124 L125 L126 L127 L128 L129 L130 L131 S168 S169 S170 L132 L133 S171 | S172 S173 S174 S175 L134 L135 S176 S177 S178 L136 L137 S179 S180 | L139 S185 S186 L140 L141 L142 L143 L144 S187 S188 L145 | S189 S190 S191 L146 L147 S192 S193 S194 S195 S196 S197 S198 L148 L149 L150 L151 L152 S199 S200 S201 | L153 L154 L155 L156 | L157 L158 S202 S203 S204 S205 S206 S207 L159 L160 S208 S209 S210 S211 S212 L161 L162 | L163 L164 L165 L166 L167 L168 L169 | L174 L175 S213 S214 S215 S216 S217 S218 L176 L177 S219 S220 S221 S222 S223 L178 L179 | S224 S225 S226 S227 | L180 L181 S236 S237 S238 S239 S240 S241 L182 L183 S242 S243 S244 S245 S246 L184 L185 | S247 S248 S249 S250 S251 S252 S253 L186 L187 S254 S255 S256 S257 S258